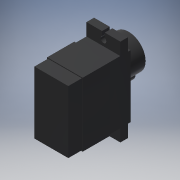
# Autodesk Inventor part: servo
Saved by Autodesk Inventor 2016 (Build 200138000, 138)
## iProperties
Created: 2016-04-27
Part Number: servo
Material: LCP Plastic
Document SubType Name: Modeling
Designer: sony
Density: 1.626 g/cm^3
Appearance: Smooth - White
Mass: 12.7174 g
Surface Area: 28.4954 cm^2
Volume: 7.82127 cm^3
Author: sony
Autodesk Inventor part; units mm, degrees
ref_plane "YZ Plane" through (0, 0, 0) normal (1, 0, 0) x (0, 1, 0)
ref_plane "XZ Plane" through (0, 0, 0) normal (0, 1, 0) x (-1, 0, 0)
ref_plane "XY Plane" through (0, 0, 0) normal (0, 0, 1) x (1, 0, 0)
sketch "Sketch1" plane through (0, 0, 0) normal (0, 1, 0) x (-1, 0, 0)
  line L0 (0, 0) -> (12.5, 0)
  line L1 (12.5, 0) -> (12.5, 23)
  line L2 (12.5, 23) -> (0, 23)
  line L3 (0, 23) -> (0, 0)
  dimension "d0" = 12.5
  dimension "d1" = 23
  constraints: 8 end point, 2 parallel, 1 horizontal, 1 perpendicular
  measures "d0" distance of L2.end L1.end
  measures "d1" distance of L1.end L0.end
extrude "Extrusion1" add sketch "Sketch1" along normal blind 23
sketch "Sketch2" plane through (0, 23, 0) normal (0, 1, 0) x (1, 0, 0)
  line L0 (0, 0) -> (-12.5, 0) projected
  line L1 (-12.5, 0) -> (-12.5, -23) projected
  line L2 (-12.5, -23) -> (0, -23) projected
  line L3 (0, -23) -> (0, 0) projected
  line L4 (0, 4.6) -> (-12.5, 4.6)
  line L5 (-12.5, 4.6) -> (-12.5, -27.6)
  line L6 (-12.5, -27.6) -> (0, -27.6)
  line L7 (0, -27.6) -> (0, 4.6)
  line L8 (0, 4.6) -> (-12.5, -27.6) construction
  line L9 (-12.5, 4.6) -> (0, -27.6) construction
  point P0 (-6.25, -11.5)
  dimension "d4" = 32.2
  constraints: 12 end point, 2 midpoint, 2 parallel, 1 horizontal, 1 perpendicular
  measures "d4" distance of L5.end L4.end
extrude "Extrusion2" add sketch "Sketch2" against normal blind 3.8 contours L0 L5 L4 L7 | L7 L6 L5 L2
sketch "Sketch3" plane through (0, 23, 0) normal (0, 1, 0) x (1, 0, 0)
  line L0 (-12.5, 4.6) -> (-12.5, -27.6) projected
  line L1 (-12.5, -27.6) -> (0, -27.6) projected
  line L2 (0, -27.6) -> (0, 4.6) projected
  line L3 (0, 4.6) -> (-12.5, 4.6) projected
  line L4 (0, -23) -> (-12.5, -23) projected
  line L5 (-12.5, 0) -> (0, 0) projected
extrude "Extrusion3" cut sketch "Sketch3" against normal blind 1 contours L3 L2 L5 L0 | L4 L2 L1 L0
sketch "Sketch4" plane through (0, 23, 0) normal (0, 1, 0) x (1, 0, 0)
  line L0 (-12.5, -23) -> (0, -23) projected
  line L1 (-6.25, -23) -> (-6.25, -16.75)
  circle A0 centre (-6.25, -16.75) radius 6.25
  dimension "d9" = 6.25
  constraints: 2 end point, 1 coincident, 1 midpoint, 1 vertical, 1 vertical alignment, 2 other
  measures "d9" distance of L1.start L1.end
extrude "Extrusion4" add sketch "Sketch4" along normal blind 5.5
sketch "Sketch5" plane through (-6.25, 28.5, 16.75) normal (0, 1, 0) x (1, 0, 0)
  circle A0 centre (0, 0) radius 6.25
  arc A1 (0, -8.95) -> (2.5, -5.72822) centre (-0.266089, -6.162672) ccw
  arc A2 (-2.5, -5.72822) -> (0, -8.95) centre (0.266089, -6.162672) ccw
  arc A3 (0, -8.95) -> (2.5, -5.72822) centre (-0.266089, -6.162672) ccw
  arc A4 (-2.5, -5.72822) -> (0, -8.95) centre (0.266089, -6.162672) ccw
  arc A5 (-2.5, -5.72822) -> (2.5, -5.72822) centre (0, 0) ccw
  line L0 (0, 0) -> (-2.287713, 0)
  arc A6 (2.5, 5.72822) -> (0, 8.95) centre (-0.266089, 6.162672) ccw
  arc A7 (0, 8.95) -> (-2.5, 5.72822) centre (0.266089, 6.162672) ccw
  arc A8 (2.5, 5.72822) -> (0, 8.95) centre (-0.266089, 6.162672) ccw
  arc A9 (0, 8.95) -> (-2.5, 5.72822) centre (0.266089, 6.162672) ccw
  arc A10 (2.5, 5.72822) -> (-2.5, 5.72822) centre (0, 0) ccw
  point P0 (6.25, 16.75)
  dimension "d14" = 2.8
  constraints: 22 point on circle, 10 centre point, 8 symmetric about line, 2 end point, 1 concentric, 1 horizontal, 5 other
  measures "d14" radius of A1
extrude "Extrusion5" add sketch "Sketch5" against normal blind 7.5 contours A0 A7 A6
sketch "Sketch6" plane through (0, 28.5, 0) normal (0, 1, 0) x (1, 0, 0)
  arc A0 (-8.75, -11.02178) -> (-3.75, -11.02178) centre (-6.25, -16.75) ccw
  circle A1 centre (-6.25, -16.75) radius 3.475
  point P0 (0, 0)
  dimension "d17" = 6.95
  constraints: 1 centre point, 1 coincident
  measures "d17" diameter of A1
extrude "Extrusion6" cut sketch "Sketch6" against normal blind 2
sketch "Sketch7" plane through (0, 28.5, 0) normal (0, 1, 0) x (1, 0, 0)
  circle A0 centre (-6.25, -16.75) radius 3.475
  arc A1 (-8.75, -11.02178) -> (-3.75, -11.02178) centre (-6.25, -16.75) ccw
  circle A2 centre (-6.25, -16.75) radius 3.5
  point P0 (0, 0)
  dimension "d20" = 7
  constraints: 1 centre point, 1 coincident
  measures "d20" diameter of A2
sketch "Sketch7 outline for Extrusion7" plane through (0, 28.5, 0) normal (0, 1, 0) x (1, 0, 0)
  circle A0 centre (-6.25, -16.75) radius 3.475
extrude "Extrusion7" cut sketch "Sketch7 outline for Extrusion7" against normal blind 2
sketch "Sketch8" plane through (0, 22, 0) normal (0, 1, 0) x (1, 0, 0)
  line L0 (0, -27.6) -> (-12.5, -27.6)
  line L1 (0, -23) -> (0, -27.6)
  line L2 (-12.5, -23) -> (0, -23)
  line L3 (-12.5, -27.6) -> (-12.5, -23)
  line L4 (-12.5, 0) -> (-12.5, 4.6)
  line L5 (0, 0) -> (-12.5, 0)
  line L6 (0, 4.6) -> (0, 0)
  line L7 (-12.5, 4.6) -> (0, 4.6)
  arc A0 (-5.75, -26.013179) -> (-6.75, -26.013179) centre (-6.25, -25.1) ccw
  arc A1 (-6.75, -27.6) -> (-5.75, -27.6) centre (-6.25, -27.6) ccw
  line L8 (0, -27.6) -> (-12.5, -27.6)
  line L9 (-5.75, -27.6) -> (-5.75, -26.013179)
  line L10 (-6.75, -27.6) -> (-6.75, -26.013179)
  line L11 (0, -23) -> (0, 0)
  line L12 (0, -11.5) -> (-20.862921, -11.5)
  arc A2 (-6.75, 3.013179) -> (-5.75, 3.013179) centre (-6.25, 2.1) ccw
  arc A3 (-5.75, 4.6) -> (-6.75, 4.6) centre (-6.25, 4.6) ccw
  line L13 (-5.75, 4.6) -> (-5.75, 3.013179)
  line L14 (-6.75, 4.6) -> (-6.75, 3.013179)
  constraints: 10 end point, 8 point on circle, 6 symmetric about line, 4 centre point, 2 point on line, 1 horizontal, 1 midpoint, 1 parallel, 1 perpendicular, 1 tangent, 2 other
extrude "Extrusion8" cut sketch "Sketch8" against normal blind 10 contours L0 L10 A0 L9 | A3 L7 | L7 L13 A2 L14
sketch "Sketch9" plane through (0, 28.5, 0) normal (0, 1, 0) x (1, 0, 0)
  circle A0 centre (-6.25, -16.75) radius 3.475
  arc A1 (-8.75, -11.02178) -> (-3.75, -11.02178) centre (-6.25, -16.75) ccw
  arc A2 (-3.75, -11.02178) -> (-6.25, -7.8) centre (-6.516089, -10.587328) ccw
  arc A3 (-6.25, -7.8) -> (-8.75, -11.02178) centre (-5.983911, -10.587328) ccw
  circle A4 centre (-6.25, -16.75) radius 2.5
  point P0 (0, 0)
  dimension "d29" = 5
  constraints: 1 centre point, 1 coincident
  measures "d29" diameter of A4
extrude "Extrusion9" add sketch "Sketch9" against normal blind 10 contours A0
sketch "Sketch10" plane through (-12.5, 0, 0) normal (-1, 0, 0) x (0, 0, 1)
  line L0 (0, 23) -> (0, 22) projected
  line L1 (0, 22) -> (-4.6, 22) projected
  line L2 (-4.6, 22) -> (-4.6, 19.2) projected
  line L3 (0, 19.2) -> (-4.6, 19.2) projected
  line L4 (0, 0) -> (0, 19.2) projected
  line L5 (0, 0) -> (23, 0) projected
  line L6 (23, 0) -> (23, 19.2) projected
  line L7 (27.6, 19.2) -> (23, 19.2) projected
  line L8 (27.6, 22) -> (27.6, 19.2) projected
  line L9 (27.6, 22) -> (23, 22) projected
  line L10 (23, 22) -> (23, 23) projected
  line L11 (16.75, 23) -> (23, 23) projected
  line L12 (0, 23) -> (16.75, 23) projected
  line L13 (0, 0) -> (0, 5)
  line L14 (0, 0) -> (0, 19.2) projected
  line L15 (0, 5) -> (23, 5)
  line L16 (23, 0) -> (23, 19.2) projected
  line L17 (0, 5) -> (0, 15)
  line L18 (0, 15) -> (23, 15)
  dimension "d32" = 5
  dimension "d33" = 10
  constraints: 8 end point, 4 point on line, 2 perpendicular
  measures "d32" distance of L4.start L13.end
  measures "d33" distance of L13.end L17.end
extrude "Extrusion11" add sketch "Sketch10" along normal blind 0.3 contours L18 L6 L15 L4
sketch "Sketch11" plane through (-12.5, 0, 23) normal (0, 0, 1) x (1, 0, 0)
  line L0 (12.5, 0) -> (12.5, 19.2) projected
  line L1 (-0.3, 5) -> (-0.3, 15) projected
  line L2 (-0.3, 15) -> (12.5, 15)
  line L3 (12.5, 15) -> (12.8, 15)
  line L4 (12.8, 15) -> (-0.3, 15)
  line L5 (-0.3, 15) -> (-0.3, 5)
  line L6 (-0.3, 5) -> (12.8, 5)
  line L7 (12.8, 5) -> (12.8, 15)
  point P0 (0, 15)
  dimension "d38" = 0.3
  constraints: 12 end point, 2 parallel, 2 perpendicular, 2 point on line, 1 horizontal
  measures "d38" distance of L2.end L3.end
extrude "Extrusion12" add sketch "Sketch11" along normal blind 0.3
sketch "Sketch12" plane through (0, 0, 23) normal (1, 0, 0) x (0, 0, -1)
  line L0 (23, 22) -> (23, 23)
  line L1 (6.25, 23) -> (23, 23)
  line L2 (0, 23) -> (6.25, 23)
  line L3 (0, 23) -> (0, 22)
  line L4 (0, 22) -> (-4.6, 22)
  line L5 (-4.6, 22) -> (-4.6, 19.2)
  line L6 (0, 19.2) -> (-4.6, 19.2)
  line L7 (0, 15) -> (0, 19.2)
  line L8 (0, 5) -> (0, 15)
  line L9 (0, 0) -> (0, 5)
  line L10 (0, 0) -> (23, 0)
  line L11 (23, 0) -> (23, 19.2)
  line L12 (27.6, 19.2) -> (23, 19.2)
  line L13 (27.6, 22) -> (27.6, 19.2)
  line L14 (27.6, 22) -> (23, 22)
  line L15 (23, 0) -> (23, 19.2)
  line L16 (-0.411339, 5) -> (23, 5)
  line L17 (23, 5) -> (23.3, 5)
  line L18 (-0.3, 15) -> (23.3, 15)
  line L19 (23.3, 15) -> (23.3, 5)
  line L20 (23.3, 5) -> (-0.3, 5)
  line L21 (-0.3, 5) -> (-0.3, 15)
  dimension "d41" = 0.3
  constraints: 12 end point, 2 parallel, 2 perpendicular, 1 horizontal, 1 point on line
  measures "d41" distance of L16.end L17.end
extrude "Extrusion13" add sketch "Sketch12" along normal blind 0.3 contours L18 L19 L17 L11 | L11 L16 L8 L18 | L8 L16 L21 L18
sketch "Sketch13" plane through (0, 0, 0) normal (0, 0, -1) x (-1, 0, 0)
  line L0 (-0.3, 5) -> (12.8, 5)
  line L1 (12.8, 5) -> (12.8, 15)
  line L2 (12.8, 15) -> (-0.3, 15)
  line L3 (-0.3, 15) -> (-0.3, 5)
  point P0 (0, 0)
  constraints: 8 end point, 2 parallel, 1 horizontal, 1 perpendicular
extrude "Extrusion14" add sketch "Sketch13" along normal blind 0.3
body "Solid1"
